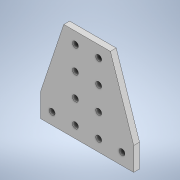
# Autodesk Inventor part: 2x1 T plate
Saved by Autodesk Inventor 2020 (Build 240168000, 168)
## iProperties
Created: 2020-01-14
Part Number: 2x1 T plate
Material: Generic
Document SubType Name: Modeling
Designer: 329817
Density: 1 g/cm^3
Appearance: Default
Author: 329817
Autodesk Inventor part; units mm, degrees
ref_plane "YZ Plane" through (0, 0, 0) normal (1, 0, 0) x (0, 1, 0)
ref_plane "XZ Plane" through (0, 0, 0) normal (0, 1, 0) x (-1, 0, 0)
ref_plane "XY Plane" through (0, 0, 0) normal (0, 0, 1) x (1, 0, 0)
sketch "Sketch1" plane through (0, 0, 0) normal (0, 0, 1) x (1, 0, 0)
  line L0 (0, 0) -> (101.6, 0)
  line L1 (101.6, 0) -> (101.6, 101.6)
  line L2 (76.2, 101.6) -> (25.4, 101.6)
  line L3 (0, 101.6) -> (0, 0)
  circle A0 centre (12.7, 12.7) radius 3.2512
  circle A1 centre (38.1, 12.7) radius 3.2512
  circle A2 centre (63.5, 12.7) radius 3.2512
  circle A3 centre (88.9, 12.7) radius 3.2512
  circle A4 centre (38.1, 38.1) radius 3.2512
  circle A5 centre (63.5, 38.1) radius 3.2512
  circle A6 centre (38.1, 63.5) radius 3.2512
  circle A7 centre (63.5, 63.5) radius 3.2512
  circle A8 centre (38.1, 88.9) radius 3.2512
  circle A9 centre (63.5, 88.9) radius 3.2512
  line L4 (25.4, 101.6) -> (0, 25.4)
  line L5 (76.2, 101.6) -> (101.6, 25.4)
  dimension "d0" = 101.6
  dimension "d1" = 101.6
  dimension "d2" = 25.4
  dimension "d3" = 25.4
  dimension "d4" = 6.5024
  dimension "d5" = 12.7
  dimension "d6" = 12.7
  dimension "d9" = 25.4
  dimension "d16" = 25.4
  dimension "d21" = 25.4
  dimension "d22" = 25.4
  constraints: 12 end point, 10 centre point, 2 horizontal, 2 parallel, 2 point on line, 1 perpendicular, 1 vertical, 18 other
  measures "d0" distance of L0.start L0.end
  measures "d1" distance of L0.end L1.end
  measures "d2" distance of L0.start L4.end
  measures "d3" distance of L0.end L5.end
  measures "d4" diameter of A0
  measures "d5" distance from line of L3 A0.centre
  measures "d6" distance from line of L0 A0.centre
  measures "d9" distance of A0.centre A1.centre
  measures "d16" distance of A1.centre A4.centre
  measures "d21" distance of L2.end L3.start
  measures "d22" distance of L2.start L1.end
extrude "Extrusion1" add sketch "Sketch1" along normal blind 6.35
body "Solid1"
